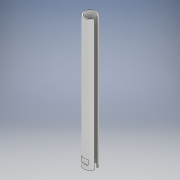
# Autodesk Inventor part: outer_sheath
Saved by Autodesk Inventor 2017 (Build 210142000, 142)
## iProperties
Created: 2018-11-30
Part Number: outer_sheath
Material: Acetal Resin, White
Document SubType Name: Modeling
Designer: ddeboer
Density: 1.425 g/cm^3
Appearance: Smooth - White
Author: ddeboer
Autodesk Inventor part; units mm, degrees
ref_plane "YZ Plane" through (0, 0, 0) normal (1, 0, 0) x (0, 1, 0)
ref_plane "XZ Plane" through (0, 0, 0) normal (0, 1, 0) x (-1, 0, 0)
sketch "Sketch1" plane through (0, 0, 0) normal (0, 0, 1) x (1, 0, 0)
  circle A0 centre (0, 0) radius 21.08
  circle A1 centre (0, 0) radius 17.35
  dimension "d0" = 42.16
  dimension "d1" = 3.73
  constraints: 2 centre point, 1 coincident
  measures "d0" diameter of A0
  measures "d1" radial gap between concentric circles of A1 A0
extrude "Extrusion1" add sketch "Sketch1" along normal blind 445
ref_plane "Work Plane1" through (0, 0, 32) normal (0, 0, 1) x (1, 0, 0)
sketch "Sketch6" plane through (0, 0, 32) normal (0, 0, 1) x (1, 0, 0)
  line L0 (11.1371, -22.214) -> (-11.1371, -22.214)
  line L1 (-11.1371, -22.214) -> (-11.1371, -18)
  line L2 (-11.1371, -18) -> (11.1371, -18)
  line L3 (11.1371, -18) -> (11.1371, -22.214)
  line L4 (0, -22.214) -> (0, -18) construction
  line L5 (0, 0) -> (0, -21.08) construction
  circle A0 centre (0, 0) radius 21.08 projected
  line L6 (0, 0) -> (6.3886, 0) construction
  line L7 (11.1371, 22.214) -> (-11.1371, 22.214)
  line L8 (-11.1371, 22.214) -> (-11.1371, 18)
  line L9 (-11.1371, 18) -> (11.1371, 18)
  line L10 (11.1371, 18) -> (11.1371, 22.214)
  line L11 (0, 22.214) -> (0, 18) construction
  point P0 (20.2483, 5.8629)
  point P1 (21.08, 0)
  point P2 (0, 21.08)
  dimension "d10" = 18
  constraints: 24 end point, 7 symmetric about line, 2 horizontal, 2 midpoint, 2 parallel, 2 perpendicular, 1 collinear, 1 point on circle
  measures "d10" distance from line of L2 L5.start
extrude "Extrusion4" cut sketch "Sketch6" against normal blind 17.5 contours L0 L1 L2 A0 L3 | A0 L2 | L9 L8 L7 L10 A0 | A0 L9
sketch "Sketch7" plane through (0, 0, 445) normal (0, 0, 1) x (1, 0, 0)
  line L0 (30, -5.75) -> (0, -5.75)
  line L1 (0, -5.75) -> (0, 5.75)
  line L2 (0, 5.75) -> (30, 5.75)
  line L3 (30, 5.75) -> (30, -5.75)
  point P0 (0, 0)
  point P1 (0, 0)
  dimension "d13" = 30
  dimension "d14" = 11.5
  constraints: 8 end point, 2 parallel, 1 coincident, 1 horizontal, 1 midpoint, 1 perpendicular
  measures "d13" distance of L1.end L2.end
  measures "d14" distance of L0.end L1.end
extrude "Extrusion5" cut sketch "Sketch7" against normal up to next
body "Solid1"
